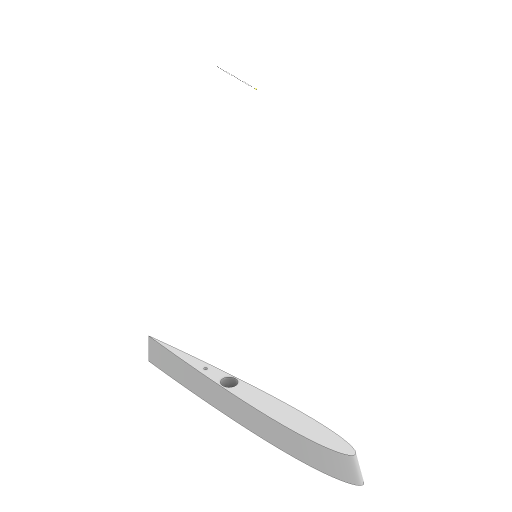
# Autodesk Inventor part: 5P.00.01.01-IB-VTP-Body-Section1
Saved by Autodesk Inventor 2024 (Build 280153000, 153)
## iProperties
Created: 2024-11-01
Part Number: 5P.00.01.01-IB-VTP-Body-Section1
Material: Generic
Document SubType Name: Modeling
Designer: inigo
Density: 1 g/cm^3
Appearance: Default
Author: inigo
Autodesk Inventor part; units mm, degrees
ref_plane "YZ Plane" through (0, 0, 0) normal (1, 0, 0) x (0, 1, 0)
ref_plane "XZ Plane" through (0, 0, 0) normal (0, 1, 0) x (-1, 0, 0)
sketch "Sketch1" plane through (0, 0, 0) normal (0, 1, 0) x (-1, 0, 0)
  spline S0 degree 4 poles (92.5, 0) (92.4441, 0.0067) (92.1719, 0.0396) (91.716, 0.0948) (90.9481, 0.186) (90.144, 0.2811) (89.1614, 0.3954) (88.0112, 0.5276) (86.6949, 0.6762) (85.2194, 0.8398) (83.5897, 1.0166) (81.8129, 1.2053) (79.8954, 1.4038) (77.8454, 1.6106) (75.6704, 1.824) (73.3795, 2.042) (70.9813, 2.2631) (68.4857, 2.4852) (65.9023, 2.7069) (63.2412, 2.926) (60.5131, 3.1407) (57.7288, 3.349) (54.8992, 3.5491) (52.0354, 3.7387) (49.1487, 3.9159) (46.2506, 4.0781) (43.3526, 4.224) (40.4658, 4.3503) (37.602, 4.456) (34.7722, 4.5382) (31.9877, 4.5959) (29.2595, 4.6265) (26.5982, 4.6291) (24.0144, 4.6026) (21.5184, 4.5458) (19.1198, 4.4584) (16.8284, 4.3403) (14.6527, 4.1916) (12.6019, 4.0129) (10.6834, 3.8054) (8.9054, 3.5701) (7.274, 3.3089) (5.7963, 3.0232) (4.477, 2.7153) (3.3214, 2.3872) (2.3326, 2.041) (1.5126, 1.6776) (0.8608, 1.2979) (0.3772, 0.8964) (0.0657, 0.4673) (-0.0448, 0) (0.0657, -0.4673) (0.3772, -0.8964) (0.8608, -1.2979) (1.5126, -1.6776) (2.3326, -2.041) (3.3214, -2.3872) (4.477, -2.7153) (5.7963, -3.0232) (7.274, -3.3089) (8.9054, -3.5701) (10.6834, -3.8054) (12.6019, -4.0129) (14.6527, -4.1916) (16.8284, -4.3403) (19.1198, -4.4584) (21.5184, -4.5458) (24.0144, -4.6026) (26.5982, -4.6291) (29.2595, -4.6265) (31.9877, -4.5959) (34.7722, -4.5382) (37.602, -4.456) (40.4658, -4.3503) (43.3526, -4.224) (46.2506, -4.0781) (49.1487, -3.9159) (52.0354, -3.7387) (54.8992, -3.5491) (57.7288, -3.349) (60.5131, -3.1407) (63.2412, -2.926) (65.9023, -2.7069) (68.4857, -2.4852) (70.9813, -2.2631) (73.3795, -2.042) (75.6704, -1.824) (77.8454, -1.6106) (79.8954, -1.4038) (81.8129, -1.2053) (83.5897, -1.0166) (85.2194, -0.8398) (86.6949, -0.6762) (88.0112, -0.5276) (89.1614, -0.3954) (90.144, -0.2811) (90.9481, -0.186) (91.716, -0.0948) (92.1719, -0.0396) (92.4441, -0.0067) (92.5, 0) knots 0 0 0 0 0 0.009356 0.014857 0.021248 0.0284 0.036221 0.044641 0.053603 0.063059 0.072965 0.083282 0.093975 0.105009 0.116353 0.127977 0.139851 0.151947 0.164237 0.176694 0.189291 0.202002 0.214801 0.227662 0.240559 0.253468 0.266361 0.279215 0.292002 0.304699 0.317279 0.329716 0.341985 0.354059 0.365912 0.377517 0.388847 0.399872 0.410565 0.420894 0.430828 0.440334 0.449378 0.457922 0.465928 0.473361 0.480192 0.48642 0.49211 0.497417 0.502583 0.50789 0.51358 0.519808 0.526639 0.534072 0.542078 0.550622 0.559666 0.569172 0.579106 0.589435 0.600128 0.611153 0.622483 0.634088 0.645941 0.658015 0.670284 0.682721 0.695301 0.707998 0.720785 0.733639 0.746532 0.759441 0.772338 0.785199 0.797998 0.810709 0.823306 0.835763 0.848053 0.860149 0.872023 0.883647 0.894991 0.906025 0.916718 0.927035 0.936941 0.946397 0.955359 0.963779 0.9716 0.978752 0.985143 0.990644 1 1 1 1 1
  point P0 (0, 0)
  point P1 (92.1353, 0.044)
  point P2 (91.6808, 0.0987)
  point P3 (91.047, 0.1742)
  point P4 (90.2363, 0.2699)
  point P5 (89.2521, 0.3846)
  point P6 (88.0983, 0.5172)
  point P7 (86.7792, 0.6662)
  point P8 (85.3002, 0.8302)
  point P9 (83.667, 1.0075)
  point P10 (81.8863, 1.1966)
  point P11 (79.9648, 1.3956)
  point P12 (77.9103, 1.6029)
  point P13 (75.7309, 1.8168)
  point P14 (73.4351, 2.0354)
  point P15 (71.032, 2.2569)
  point P16 (68.5311, 2.4796)
  point P17 (65.9423, 2.7016)
  point P18 (63.2757, 2.9211)
  point P19 (60.542, 3.1362)
  point P20 (57.7519, 3.3449)
  point P21 (54.9164, 3.5452)
  point P22 (52.0467, 3.7351)
  point P23 (49.154, 3.9123)
  point P24 (46.25, 4.0747)
  point P25 (43.346, 4.2203)
  point P26 (40.4533, 4.3467)
  point P27 (37.5836, 4.4519)
  point P28 (34.7481, 4.5339)
  point P29 (31.958, 4.5909)
  point P30 (29.2243, 4.6209)
  point P31 (26.5577, 4.6228)
  point P32 (23.9689, 4.5952)
  point P33 (21.468, 4.5373)
  point P34 (19.0649, 4.4486)
  point P35 (16.7691, 4.3289)
  point P36 (14.5897, 4.1784)
  point P37 (12.5352, 3.9977)
  point P38 (10.6137, 3.7877)
  point P39 (8.833, 3.5496)
  point P40 (7.1998, 3.285)
  point P41 (5.7208, 2.9953)
  point P42 (4.4017, 2.6827)
  point P43 (3.2479, 2.3489)
  point P44 (2.2637, 1.996)
  point P45 (1.453, 1.6255)
  point P46 (0.8192, 1.2394)
  point P47 (0.3647, 0.839)
  point P48 (0.0913, 0.4256)
  point P49 (0, 0)
  point P50 (0.0913, -0.4256)
  point P51 (0.3647, -0.839)
  point P52 (0.8192, -1.2394)
  point P53 (1.453, -1.6255)
  point P54 (2.2637, -1.996)
  point P55 (3.2479, -2.3489)
  point P56 (4.4017, -2.6827)
  point P57 (5.7208, -2.9953)
  point P58 (7.1998, -3.285)
  point P59 (8.833, -3.5496)
  point P60 (10.6137, -3.7877)
  point P61 (12.5352, -3.9977)
  point P62 (14.5897, -4.1784)
  point P63 (16.7691, -4.3289)
  point P64 (19.0649, -4.4486)
  point P65 (21.468, -4.5373)
  point P66 (23.9689, -4.5952)
  point P67 (26.5577, -4.6228)
  point P68 (29.2243, -4.6209)
  point P69 (31.958, -4.5909)
  point P70 (34.7481, -4.5339)
  point P71 (37.5836, -4.4519)
  point P72 (40.4533, -4.3467)
  point P73 (43.346, -4.2203)
  point P74 (46.25, -4.0747)
  point P75 (49.154, -3.9123)
  point P76 (52.0467, -3.7351)
  point P77 (54.9164, -3.5452)
  point P78 (57.7519, -3.3449)
  point P79 (60.542, -3.1362)
  point P80 (63.2757, -2.9211)
  point P81 (65.9423, -2.7016)
  point P82 (68.5311, -2.4796)
  point P83 (71.032, -2.2569)
  point P84 (73.4351, -2.0354)
  point P85 (75.7309, -1.8168)
  point P86 (77.9103, -1.6029)
  point P87 (79.9648, -1.3956)
  point P88 (81.8863, -1.1966)
  point P89 (83.667, -1.0075)
  point P90 (85.3002, -0.8302)
  point P91 (86.7792, -0.6662)
  point P92 (88.0983, -0.5172)
  point P93 (89.2521, -0.3846)
  point P94 (90.2363, -0.2699)
  point P95 (91.047, -0.1742)
  point P96 (91.6808, -0.0987)
  point P97 (92.1353, -0.044)
  point P98 (92.4087, -0.011)
  constraints: 101 other
ref_plane "Work Plane1" through (-31.958, 0, -4.5909) normal (0, 1, 0) x (0, 0, 1)
ref_plane "Work Plane2" through (-31.958, -250, -4.5909) normal (0, 1, 0) x (0, 0, 1)
sketch "Sketch2" plane through (-31.958, -250, -4.5909) normal (0, 1, 0) x (0, 0, 1)
  spline S0 degree 4 poles (4.591, -60.542) (4.6044, -60.4303) (4.6702, -59.8859) (4.7806, -58.9739) (4.963, -57.4381) (5.1532, -55.83) (5.3819, -53.8647) (5.6462, -51.5645) (5.9434, -48.9317) (6.2707, -45.9809) (6.6243, -42.7214) (7.0016, -39.1678) (7.3987, -35.3328) (7.8122, -31.2328) (8.239, -26.8828) (8.6751, -22.301) (9.1173, -17.5046) (9.5614, -12.5134) (10.0049, -7.3465) (10.4429, -2.0244) (10.8723, 3.4317) (11.2889, 9.0003) (11.6893, 14.6597) (12.0683, 20.3872) (12.4227, 26.1606) (12.7472, 31.9567) (13.0389, 37.7528) (13.2915, 43.5263) (13.503, 49.254) (13.6673, 54.9136) (13.7827, 60.4825) (13.8439, 65.9391) (13.8493, 71.2617) (13.7962, 76.4292) (13.6826, 81.4211) (13.5079, 86.2184) (13.2716, 90.8013) (12.9743, 95.1526) (12.6167, 99.2542) (12.2019, 103.0912) (11.7311, 106.6472) (11.2088, 109.9099) (10.6373, 112.8655) (10.0216, 115.504) (9.3654, 117.8151) (8.673, 119.7928) (7.9462, 121.4327) (7.1867, 122.7364) (6.3839, 123.7036) (5.5256, 124.3265) (4.591, 124.5476) (3.6564, 124.3265) (2.7981, 123.7036) (1.9953, 122.7364) (1.2358, 121.4327) (0.509, 119.7928) (-0.1834, 117.8151) (-0.8396, 115.504) (-1.4553, 112.8655) (-2.0268, 109.9099) (-2.5491, 106.6472) (-3.0199, 103.0912) (-3.4347, 99.2542) (-3.7923, 95.1526) (-4.0896, 90.8013) (-4.3259, 86.2184) (-4.5006, 81.4211) (-4.6142, 76.4292) (-4.6673, 71.2617) (-4.6619, 65.9391) (-4.6007, 60.4825) (-4.4853, 54.9136) (-4.321, 49.254) (-4.1095, 43.5263) (-3.8569, 37.7528) (-3.5652, 31.9567) (-3.2407, 26.1606) (-2.8863, 20.3872) (-2.5073, 14.6597) (-2.1069, 9.0003) (-1.6903, 3.4317) (-1.2609, -2.0244) (-0.8229, -7.3465) (-0.3794, -12.5134) (0.0647, -17.5046) (0.5069, -22.301) (0.943, -26.8828) (1.3698, -31.2328) (1.7833, -35.3328) (2.1804, -39.1678) (2.5577, -42.7214) (2.9113, -45.9809) (3.2386, -48.9317) (3.5358, -51.5645) (3.8001, -53.8647) (4.0288, -55.83) (4.219, -57.4381) (4.4014, -58.9739) (4.5118, -59.8859) (4.5776, -60.4303) (4.591, -60.542) knots 0 0 0 0 0 0.009356 0.014857 0.021248 0.0284 0.036221 0.044641 0.053603 0.063059 0.072965 0.083282 0.093975 0.105009 0.116353 0.127977 0.139851 0.151947 0.164237 0.176694 0.189291 0.202002 0.214801 0.227662 0.240559 0.253468 0.266361 0.279215 0.292002 0.304699 0.317279 0.329716 0.341985 0.354059 0.365912 0.377517 0.388847 0.399872 0.410565 0.420894 0.430828 0.440334 0.449378 0.457922 0.465928 0.473361 0.480192 0.48642 0.49211 0.497417 0.502583 0.50789 0.51358 0.519808 0.526639 0.534072 0.542078 0.550622 0.559666 0.569172 0.579106 0.589435 0.600128 0.611153 0.622483 0.634088 0.645941 0.658015 0.670284 0.682721 0.695301 0.707998 0.720785 0.733639 0.746532 0.759441 0.772338 0.785199 0.797998 0.810709 0.823306 0.835763 0.848053 0.860149 0.872023 0.883647 0.894991 0.906025 0.916718 0.927035 0.936941 0.946397 0.955359 0.963779 0.9716 0.978752 0.985143 0.990644 1 1 1 1 1
  point P0 (4.5909, 31.958)
  point P1 (4.6791, -59.8125)
  point P2 (4.7884, -58.9036)
  point P3 (4.9394, -57.636)
  point P4 (5.1308, -56.0147)
  point P5 (5.3602, -54.0463)
  point P6 (5.6253, -51.7386)
  point P7 (5.9234, -49.1003)
  point P8 (6.2514, -46.1423)
  point P9 (6.606, -42.876)
  point P10 (6.9842, -39.3145)
  point P11 (7.3823, -35.4715)
  point P12 (7.7969, -31.3627)
  point P13 (8.2246, -27.0037)
  point P14 (8.6617, -22.4122)
  point P15 (9.1048, -17.6059)
  point P16 (9.5501, -12.6042)
  point P17 (9.9943, -7.4266)
  point P18 (10.4333, -2.0935)
  point P19 (10.8634, 3.374)
  point P20 (11.2808, 8.9542)
  point P21 (11.6815, 14.6252)
  point P22 (12.0611, 20.3646)
  point P23 (12.4156, 26.1499)
  point P24 (12.7404, 31.958)
  point P25 (13.0316, 37.7661)
  point P26 (13.2843, 43.5514)
  point P27 (13.4949, 49.2908)
  point P28 (13.6588, 54.9618)
  point P29 (13.7727, 60.542)
  point P30 (13.8329, 66.0095)
  point P31 (13.8366, 71.3427)
  point P32 (13.7814, 76.5202)
  point P33 (13.6656, 81.5219)
  point P34 (13.4882, 86.3282)
  point P35 (13.2488, 90.9197)
  point P36 (12.9478, 95.2787)
  point P37 (12.5863, 99.3875)
  point P38 (12.1664, 103.2305)
  point P39 (11.6902, 106.792)
  point P40 (11.1609, 110.0583)
  point P41 (10.5817, 113.0163)
  point P42 (9.9564, 115.6546)
  point P43 (9.2889, 117.9623)
  point P44 (8.5829, 119.9307)
  point P45 (7.842, 121.552)
  point P46 (7.0698, 122.8196)
  point P47 (6.269, 123.7285)
  point P48 (5.4422, 124.2754)
  point P49 (4.591, 124.458)
  point P50 (3.7398, 124.2754)
  point P51 (2.9131, 123.7285)
  point P52 (2.1122, 122.8196)
  point P53 (1.34, 121.552)
  point P54 (0.5991, 119.9307)
  point P55 (-0.1069, 117.9623)
  point P56 (-0.7744, 115.6546)
  point P57 (-1.3997, 113.0163)
  point P58 (-1.9789, 110.0583)
  point P59 (-2.5082, 106.792)
  point P60 (-2.9844, 103.2305)
  point P61 (-3.4043, 99.3875)
  point P62 (-3.7658, 95.2787)
  point P63 (-4.0668, 90.9197)
  point P64 (-4.3062, 86.3282)
  point P65 (-4.4836, 81.5219)
  point P66 (-4.5994, 76.5202)
  point P67 (-4.6546, 71.3427)
  point P68 (-4.6509, 66.0095)
  point P69 (-4.5907, 60.542)
  point P70 (-4.4768, 54.9618)
  point P71 (-4.3129, 49.2908)
  point P72 (-4.1023, 43.5514)
  point P73 (-3.8496, 37.7661)
  point P74 (-3.5584, 31.958)
  point P75 (-3.2336, 26.1499)
  point P76 (-2.8791, 20.3646)
  point P77 (-2.4995, 14.6252)
  point P78 (-2.0988, 8.9542)
  point P79 (-1.6814, 3.374)
  point P80 (-1.2513, -2.0935)
  point P81 (-0.8123, -7.4266)
  point P82 (-0.3681, -12.6042)
  point P83 (0.0772, -17.6059)
  point P84 (0.5203, -22.4122)
  point P85 (0.9574, -27.0037)
  point P86 (1.3851, -31.3627)
  point P87 (1.7997, -35.4715)
  point P88 (2.1978, -39.3145)
  point P89 (2.576, -42.876)
  point P90 (2.9306, -46.1423)
  point P91 (3.2586, -49.1003)
  point P92 (3.5567, -51.7386)
  point P93 (3.8218, -54.0463)
  point P94 (4.0512, -56.0147)
  point P95 (4.2426, -57.636)
  point P96 (4.3936, -58.9036)
  point P97 (4.5029, -59.8125)
  point P98 (4.569, -60.3594)
  constraints: 101 other
loft "Loft1" add profiles "Sketch2", "Sketch1"
sketch "Sketch4" plane through (-31.958, 0, -4.5909) normal (0, 1, 0) x (0, 0, 1)
  line L0 (4.5909, -1.5651) -> (4.5909, 34.9925)
  point P0 (4.5909, 31.958)
  constraints: 2 end point, 1 vertical
ref_plane "Work Plane3" through (-33.5232, 0, 0) normal (0, 0, 1) x (1, 0, 0)
sketch "Sketch5" plane through (-33.5232, 0, 0) normal (0, 0, 1) x (1, 0, 0)
  line L0 (-58.9768, 0) -> (33.5232, 0) projected
  line L1 (-58.9769, -250) -> (-58.9768, 0) projected
  line L2 (-58.9769, -250) -> (126.0231, -250) projected
  line L3 (-58.9769, -250) -> (-58.9768, 0) projected
  line L4 (-58.9768, 0) -> (33.5232, 0) projected
  line L5 (-58.9768, -18.985) -> (-9.4768, -18.985)
  line L6 (-9.4768, -18.985) -> (-9.4768, -231.015)
  line L7 (-9.4768, -231.015) -> (-58.9768, -231.015)
  line L8 (-58.9768, -231.015) -> (-58.9768, -18.985)
  dimension "d11" = 49.5
  dimension "d12" = 212.03
  dimension "d13" = 18.985
  constraints: 8 end point, 2 parallel, 1 horizontal, 1 perpendicular, 1 point on line
  measures "d11" distance of L5.start L5.end
  measures "d12" distance of L5.end L6.end
  measures "d13" distance between parallel lines of L0 L5
split body "Split1" sketch "Sketch5" result two bodies curves L6 L7 L8 L5 first body at (-32.8761, -207.6767, -5.3253)
sketch "Sketch6" plane through (-43, -231.015, 5.0629) normal (0, 1, 0) x (1, 0, 0)
  line L0 (0, 9.4331) -> (0, 0.6928) projected
  line L1 (0, 10.1256) -> (0, 0) projected
  line L2 (0, 14.4041) -> (6.031, 14.4041)
  line L3 (6.031, 14.4041) -> (6.031, -3.6982)
  line L4 (6.031, -3.6982) -> (0, -3.6982)
  line L5 (0, -3.6982) -> (0, 14.4041)
  point P0 (43, 5.0629)
  dimension "d25" = 6.031
  constraints: 8 end point, 2 parallel, 1 horizontal, 1 perpendicular
  measures "d25" distance of L3.end L4.end
sketch "Sketch7" plane through (-43, -18.985, -4.3701) normal (0, -1, 0) x (1, 0, 0)
  line L0 (0, 0) -> (0, 8.7403) projected
  line L1 (0, -4.2658) -> (4.936, -4.2658)
  line L2 (4.936, -4.2658) -> (4.936, 11.3897)
  line L3 (4.936, 11.3897) -> (0, 11.3897)
  line L4 (0, 11.3897) -> (0, -4.2658)
  point P0 (43, 4.3701)
  dimension "d26" = 4.936
  constraints: 8 end point, 2 parallel, 1 horizontal, 1 perpendicular
  measures "d26" distance of L3.end L2.end
loft "Loft2" cut profiles "Sketch7", "Sketch6"
sketch "Sketch8" plane through (-30.8333, -231.015, 0) normal (0, 1, 0) x (1, 0, 0.0002312)
  circle A0 centre (-12.6667, 0) radius 1.25
  point P0 (30.8333, 0.0071)
  point P1 (-61.6667, -0.0144)
  dimension "d18" = 2.5
  dimension "d32" = 49
  constraints: 1 centre point
  measures "d18" diameter of A0
  measures "d32" distance of point (-61.667, -0.014) A0.centre
extrude "Extrusion1" cut sketch "Sketch8" along normal blind 210 and the other way blind 20 bodies 2
sketch "Sketch9" plane through (0, 0, 0) normal (0, 0, 1) x (1, 0, 0)
  line L0 (-138.2387, -231.015) -> (187.2192, -231.015)
  point P0 (0, 0)
  dimension "d27" = 231.015
  constraints: 2 end point, 1 horizontal
  measures "d27" distance from line of point (0, 0) L0
split body "Split2" sketch "Sketch9" result one side removed bodies 2 curves L0 removed pieces at (-15.6753, -222.1826, -6.5801)
sketch "Sketch10" plane through (-31.958, -250, -4.5909) normal (0, 1, 0) x (0, 0, 1)
  circle A0 centre (4.5909, 8.833) radius 5.5
  point P0 (4.5909, 31.958)
  dimension "d28" = 11
  dimension "d29" = 69.375
  constraints: 1 centre point, 1 other
  measures "d28" diameter of A0
  measures "d29" distance of point (4.591, -60.542) A0.centre
extrude "Extrusion2" cut sketch "Sketch10" along normal through all bodies 2
equation "\"d11\" = rudWidth"
equation "\"d12\" = rudLength"
equation "\"d13\" = rudHingeSeatLength"
equation "\"rudHingeSeatLength\" = 18.985"
equation "\"rudLength\" = vtpLength - 2 * rudHingeSeatLength"
equation "\"rudWidth\" = 49.5"
equation "\"rootChord\" = 185"
equation "\"vtpLength\" = 250"
body "Solid2"
body "Solid3"
